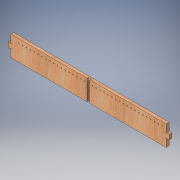
# Autodesk Inventor part: shelf back 2
Saved by Autodesk Inventor 2016 (Build 200138000, 138)
## iProperties
Created: 2017-03-13
Part Number: shelf back 2
Material: Wood (Birch)
Document SubType Name: Modeling
Designer: jwillauer
Density: 0.55 g/cm^3
Appearance: Birch - Natural Polished
Author: jwillauer
Autodesk Inventor part; units mm, degrees
ref_plane "YZ Plane" through (0, 0, 0) normal (1, 0, 0) x (0, 1, 0)
ref_plane "XZ Plane" through (0, 0, 0) normal (0, 1, 0) x (-1, 0, 0)
ref_plane "XY Plane" through (0, 0, 0) normal (0, 0, 1) x (1, 0, 0)
sketch "Sketch1" plane through (0, 0, 0) normal (0, 0, 1) x (1, 0, 0)
  line L0 (-599.9626, 113.7827) -> (416.0374, 113.7827)
  line L1 (416.0374, -19.8213) -> (-599.9626, -19.8213)
  line L2 (-599.9626, 62.9827) -> (-618.7586, 62.9827)
  line L3 (-618.7586, 62.9827) -> (-618.7586, 30.9787)
  line L4 (-618.7586, 30.9787) -> (-599.9626, 30.9787)
  line L5 (416.0374, 62.9827) -> (434.8334, 62.9827)
  line L6 (434.8334, 62.9827) -> (434.8334, 30.9787)
  line L7 (434.8334, 30.9787) -> (416.0374, 30.9787)
  line L8 (-599.9626, -19.8213) -> (-599.9626, 30.9787)
  line L9 (-599.9626, 62.9827) -> (-599.9626, 113.7827)
  line L10 (416.0374, 113.7827) -> (416.0374, 62.9827)
  line L11 (416.0374, 30.9787) -> (416.0374, -19.8213)
  point P0 (0, 0)
  dimension "d0" = 133.604
  dimension "d1" = 1016
  dimension "d2" = 18.796
  dimension "d3" = 18.796
  dimension "d4" = 18.796
  dimension "d5" = 18.796
  dimension "d6" = 50.8
  dimension "d7" = 50.8
  dimension "d8" = 50.8
  dimension "d9" = 50.8
  constraints: 24 end point, 8 perpendicular, 5 parallel, 3 horizontal
  measures "d0" distance between parallel lines of L0 L1
  measures "d1" distance of L0.start L0.end
  measures "d2" distance of L2.start L2.end
  measures "d3" distance of L3.end L4.end
  measures "d4" distance of L5.start L5.end
  measures "d5" distance of L6.end L7.end
  measures "d6" distance between parallel lines of L0 L2
  measures "d7" distance between parallel lines of L1 L4
  measures "d8" distance between parallel lines of L0 L5
  measures "d9" distance of L7.end L1.start
extrude "Extrusion1" add sketch "Sketch1" along normal blind 18.796
sketch "Sketch2" plane through (0, 0, 18.796) normal (0, 0, 1) x (1, 0, 0)
  line L0 (416.0374, 113.7827) -> (-599.9626, 113.7827) projected
  line L1 (-91.9626, 113.7827) -> (-91.9626, -19.8213)
  line L2 (416.0374, -19.8213) -> (-599.9626, -19.8213) projected
  line L3 (-101.3606, 113.7827) -> (-101.3606, -19.8213)
  line L4 (-82.5646, 113.7827) -> (-82.5646, -19.8213)
  line L5 (-101.3606, 113.7827) -> (-82.5646, 113.7827)
  line L6 (-101.3606, -19.8213) -> (-82.5646, -19.8213)
  point P0 (0, 0)
  dimension "d12" = 9.398
  dimension "d13" = 9.398
  constraints: 10 end point, 2 midpoint, 2 parallel, 1 collinear, 1 perpendicular
  measures "d12" distance between parallel lines of L1 L3
  measures "d13" distance between parallel lines of L1 L4
extrude "Extrusion2" cut sketch "Sketch2" against normal blind 9.398
sketch "Sketch3" plane through (0, 0, 18.796) normal (0, 0, 1) x (1, 0, 0)
  line L0 (-599.9626, 113.7827) -> (-599.9626, 62.9827) projected
  line L1 (-599.9626, 113.7827) -> (416.0374, 113.7827) projected
  point P0 (0, 0)
  point P1 (-549.1626, 88.3827)
  point P2 (-523.7626, 88.3827)
  point P3 (-498.3626, 88.3827)
  point P4 (-472.9626, 88.3827)
  point P5 (-447.5626, 88.3827)
  point P6 (-422.1626, 88.3827)
  point P7 (-396.7626, 88.3827)
  point P8 (-371.3626, 88.3827)
  point P9 (-345.9626, 88.3827)
  point P10 (-320.5626, 88.3827)
  point P11 (-295.1626, 88.3827)
  point P12 (-269.7626, 88.3827)
  point P13 (-244.3626, 88.3827)
  point P14 (-218.9626, 88.3827)
  point P15 (-193.5626, 88.3827)
  point P16 (-168.1626, 88.3827)
  point P17 (-142.7626, 88.3827)
  point P18 (-117.3626, 88.3827)
  point P19 (-91.9626, 88.3827)
  point P20 (-66.5626, 88.3827)
  point P21 (-41.1626, 88.3827)
  point P22 (-15.7626, 88.3827)
  point P23 (9.6374, 88.3827)
  point P24 (35.0374, 88.3827)
  point P25 (60.4374, 88.3827)
  point P26 (85.8374, 88.3827)
  point P27 (111.2374, 88.3827)
  point P28 (136.6374, 88.3827)
  point P29 (162.0374, 88.3827)
  point P30 (187.4374, 88.3827)
  point P31 (212.8374, 88.3827)
  point P32 (238.2374, 88.3827)
  point P33 (263.6374, 88.3827)
  point P34 (289.0374, 88.3827)
  point P35 (314.4374, 88.3827)
  point P36 (339.8374, 88.3827)
  point P37 (365.2374, 88.3827)
  point P38 (390.6374, 88.3827)
  dimension "d16" = 50.8
  dimension "d17" = 25.4
  dimension "d20" = 25.4
  constraints: 1 horizontal, 37 other
  measures "d16" distance from line of L0 point (-549.163, 88.383)
  measures "d17" distance from line of L1 point (-549.163, 88.383)
  measures "d20" distance of point (-549.163, 88.383) point (-523.763, 88.383)
hole "Hole1" at (-549.1626, 88.3827, 18.796) at (-523.7626, 88.3827, 18.796) at (-498.3626, 88.3827, 18.796) at (-472.9626, 88.3827, 18.796) at (-447.5626, 88.3827, 18.796) at (-422.1626, 88.3827, 18.796) at (-396.7626, 88.3827, 18.796) at (-371.3626, 88.3827, 18.796) at (-345.9626, 88.3827, 18.796) at (-320.5626, 88.3827, 18.796) at (-295.1626, 88.3827, 18.796) at (-269.7626, 88.3827, 18.796) at (-244.3626, 88.3827, 18.796) at (-218.9626, 88.3827, 18.796) at (-193.5626, 88.3827, 18.796) at (-168.1626, 88.3827, 18.796) at (-142.7626, 88.3827, 18.796) at (-117.3626, 88.3827, 18.796) at (-91.9626, 88.3827, 18.796) at (-66.5626, 88.3827, 18.796) at (-41.1626, 88.3827, 18.796) at (-15.7626, 88.3827, 18.796) at (9.6374, 88.3827, 18.796) at (35.0374, 88.3827, 18.796) at (60.4374, 88.3827, 18.796) at (85.8374, 88.3827, 18.796) at (111.2374, 88.3827, 18.796) at (136.6374, 88.3827, 18.796) at (162.0374, 88.3827, 18.796) at (187.4374, 88.3827, 18.796) at (212.8374, 88.3827, 18.796) at (238.2374, 88.3827, 18.796) at (263.6374, 88.3827, 18.796) at (289.0374, 88.3827, 18.796) at (314.4374, 88.3827, 18.796) at (339.8374, 88.3827, 18.796) at (365.2374, 88.3827, 18.796) at (390.6374, 88.3827, 18.796) direction (0, 0, -1) diameter 6.35 end through all
sketch "Sketch4" plane through (0, 0, 18.796) normal (0, 0, 1) x (1, 0, 0)
  line L0 (-618.7586, 62.9827) -> (-599.9626, 62.9827) projected
  line L1 (-618.7586, 30.9787) -> (-599.9626, 30.9787) projected
  line L2 (416.0374, 62.9827) -> (434.8334, 62.9827) projected
  point P0 (0, 0)
  point P1 (416.0374, 30.9787)
hole "Hole2" at (-599.9626, 62.9827, 18.796) at (-599.9626, 30.9787, 18.796) at (416.0374, 62.9827, 18.796) at (416.0374, 30.9787, 18.796) direction (0, 0, -1) diameter 6.35 end through all
body "Solid1"
